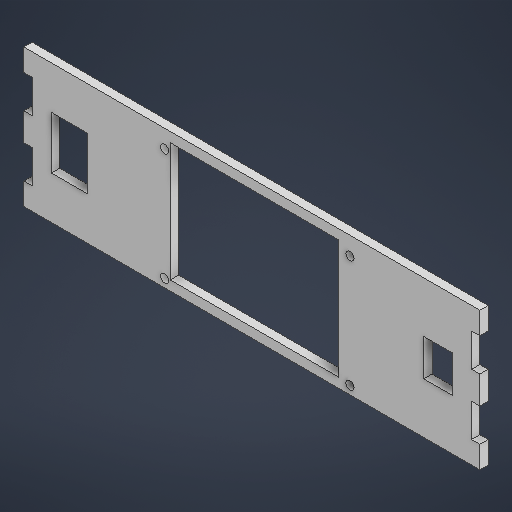
# Autodesk Inventor part: pantallaSoport
Saved by Autodesk Inventor 2026 (Build 300175000, 175)
## iProperties
Created: 2026-04-21
Part Number: pantallaSoport
Material: Generic
Document SubType Name: Modeling
Designer: juana
Density: 1 g/cm^3
Appearance: Default
Author: juana
Autodesk Inventor part; units mm, degrees
ref_plane "YZ Plane" through (0, 0, 0) normal (1, 0, 0) x (0, 1, 0)
ref_plane "XZ Plane" through (0, 0, 0) normal (0, 1, 0) x (-1, 0, 0)
ref_plane "XY Plane" through (0, 0, 0) normal (0, 0, 1) x (1, 0, 0)
sketch "Sketch1" plane through (0, 0, 0) normal (0, 0, 1) x (1, 0, 0)
  line L0 (0, 0) -> (165, 0)
  line L1 (165, 0) -> (165, 50)
  line L2 (165, 50) -> (0, 50)
  line L3 (0, 50) -> (0, 0)
  line L4 (0, 50) -> (3, 50)
  line L5 (3, 50) -> (3, 46.5)
  line L6 (3, 46.5) -> (0, 46.5)
  line L7 (0, 46.5) -> (0, 50)
  line L8 (0, 0) -> (3, 0)
  line L9 (3, 0) -> (3, 3.5)
  line L10 (3, 3.5) -> (0, 3.5)
  line L11 (0, 3.5) -> (0, 0)
  line L12 (82.5, 0) -> (82.5, 50) construction
  line L13 (162, 50) -> (162, 46.5)
  line L14 (162, 46.5) -> (165, 46.5)
  line L15 (162, 0) -> (162, 3.5)
  line L16 (162, 3.5) -> (165, 3.5)
  line L17 (44, 46.5) -> (121, 46.5) construction
  line L18 (121, 46.5) -> (121, 3.5) construction
  line L19 (121, 3.5) -> (44, 3.5) construction
  line L20 (44, 3.5) -> (44, 46.5) construction
  line L21 (53, 46.5) -> (114, 46.5)
  line L22 (114, 46.5) -> (114, 3.5)
  line L23 (114, 3.5) -> (53, 3.5)
  line L24 (53, 3.5) -> (53, 46.5)
  line L25 (3, 0) -> (0, 0)
  line L26 (0, 0) -> (0, 8)
  line L27 (0, 8) -> (3, 8)
  line L28 (3, 8) -> (3, 0)
  line L29 (0, 50) -> (3, 50)
  line L30 (3, 50) -> (3, 42)
  line L31 (3, 42) -> (0, 42)
  line L32 (0, 42) -> (0, 50)
  line L33 (0, 42) -> (3, 42)
  line L34 (3, 42) -> (3, 30)
  line L35 (3, 30) -> (0, 30)
  line L36 (0, 30) -> (0, 42)
  line L37 (3, 8) -> (0, 8)
  line L38 (0, 8) -> (0, 20)
  line L39 (0, 20) -> (3, 20)
  line L40 (3, 20) -> (3, 8)
  line L41 (165, 8) -> (162, 8)
  line L42 (162, 42) -> (165, 42)
  line L43 (162, 42) -> (162, 30)
  line L44 (162, 30) -> (165, 30)
  line L45 (165, 20) -> (162, 20)
  line L46 (162, 20) -> (162, 8)
  point P0 (1.5, 25)
  point P1 (0, 25)
  point P2 (1.5, 3.5)
  point P3 (44, 25)
  point P4 (82.5, 46.5)
  point P5 (1.5, 46.5)
  point P6 (119, 5.5)
  point P7 (119, 44.5)
  point P8 (50.5, 44.5)
  point P9 (50.5, 5.5)
  point P10 (0, 46.5)
  point P11 (0, 3.5)
  point P12 (165, 20)
  point P13 (165, 30)
  point P14 (165, 42)
  dimension "d0" = 165
  dimension "d1" = 50
  dimension "d2" = 3
  dimension "d4" = 21.5
  dimension "d5" = 21.5
  dimension "d6" = 77
  dimension "d7" = 61
  dimension "d8" = 9
  dimension "d9" = 2
  dimension "d10" = 2
  dimension "d11" = 2
  dimension "d12" = 6.5
  dimension "d13" = 2
  dimension "d34" = 8
  dimension "d35" = 8
  dimension "d36" = 12
  dimension "d37" = 12
  constraints: 94 end point, 18 parallel, 15 symmetric about line, 9 horizontal, 9 perpendicular, 7 midpoint, 7 vertical alignment, 6 horizontal alignment, 2 point on line
  measures "d0" distance of L1.end L2.end
  measures "d1" distance of L0.end L1.end
  measures "d2" distance of L5.end L6.end
  measures "d4" distance from line of L10 point (1.5, 25)
  measures "d5" distance from line of L6 point (1.5, 25)
  measures "d6" distance of L17.start L17.end
  measures "d7" distance of L21.start L21.end
  measures "d8" distance between parallel lines of L20 L24
  measures "d9" distance from line of L19 point (119, 5.5)
  measures "d10" distance from line of L17 point (119, 44.5)
  measures "d11" distance from line of L18 point (119, 44.5)
  measures "d12" distance from line of L20 point (50.5, 44.5)
  measures "d13" distance from line of L19 point (50.5, 5.5)
  measures "d34" distance of L27.end L8.end
  measures "d35" distance of L29.end L30.end
  measures "d36" distance of L33.end L34.end
  measures "d37" distance of L39.end L27.end
extrude "Extrusion1" add sketch "Sketch1" along normal blind 3 contours L3 L10 L9 L0 | L9 L28 L40 L39 L3 L35 L34 L30 L5 L2 L13 L14 L1 L42 L43 L44 L45 L46 L41 L16 L15 L0 | L3 L27 L28 L10 | L15 L16 L1 L0 | L3 L6 L30 L31 | L3 L2 L5 L6 | L14 L13 L2 L1
sketch "Sketch2" plane through (0, 0, 3) normal (0, 0, 1) x (1, 0, 0)
  line L0 (53, 46.5) -> (114, 46.5) projected
  line L1 (44, 46.5) -> (121, 46.5)
  line L2 (121, 46.5) -> (121, 0)
  line L3 (121, 0) -> (44, 0)
  line L4 (44, 0) -> (44, 46.5)
  line L5 (165, 50) -> (0, 50) projected
  line L6 (0, 8) -> (0, 0) projected
  point P0 (50.92, 43.5)
  point P1 (50.92, 3)
  point P2 (82.5, 46.5)
  point P3 (82.5, 50)
  point P4 (113, 50)
  point P5 (3, 50)
  point P6 (44, 23.25)
  point P7 (0, 4)
  point P8 (0, 46.5)
  point P9 (0, 3.5)
  point P10 (118, 43.5)
  point P11 (118, 3)
  dimension "d17" = 77
  dimension "d18" = 3
  dimension "d19" = 3
  dimension "d20" = 3
  dimension "d28" = 6.92
  constraints: 8 end point, 4 midpoint, 3 horizontal alignment, 3 vertical alignment, 2 parallel, 1 horizontal, 1 perpendicular, 1 point on line
  measures "d17" distance between parallel lines of L2 L4
  measures "d18" distance from line of L1 point (118, 43.5)
  measures "d19" distance from line of L3 point (118, 3)
  measures "d20" distance from line of L2 point (118, 3)
  measures "d28" distance from line of L4 point (50.92, 3)
hole "Hole1" at (50.92, 43.5, 3) at (50.92, 3, 3) at (118, 3, 3) at (118, 43.5, 3) direction (0, 0, -1) diameter 3 end through all
sketch "Sketch3" plane through (0, 0, 3) normal (0, 0, 1) x (1, 0, 0)
  line L0 (10, 34.5) -> (23, 34.5)
  line L1 (23, 34.5) -> (23, 15.5)
  line L2 (23, 15.5) -> (10, 15.5)
  line L3 (10, 15.5) -> (10, 34.5)
  line L4 (0, 8) -> (0, 0) construction
  line L5 (144.7, 31.65) -> (155, 31.65)
  line L6 (155, 31.65) -> (155, 18.35)
  line L7 (155, 18.35) -> (144.7, 18.35)
  line L8 (144.7, 18.35) -> (144.7, 31.65)
  line L9 (165, 20) -> (165, 30) projected
  line L10 (0, 30) -> (0, 20) projected
  point P0 (10, 25)
  point P1 (0, 46.5)
  point P2 (165, 25)
  point P3 (0, 25)
  point P4 (144.7, 25)
  dimension "d29" = 19
  dimension "d30" = 13
  dimension "d31" = 10
  dimension "d38" = 10.3
  dimension "d39" = 13.3
  dimension "d40" = 10
  constraints: 16 end point, 4 midpoint, 4 parallel, 2 horizontal, 2 horizontal alignment, 2 perpendicular
  measures "d29" distance of L2.end L0.start
  measures "d30" distance of L1.end L2.end
  measures "d31" distance between parallel lines of L4 L3
  measures "d38" distance of L5.start L5.end
  measures "d39" distance of L5.end L6.end
  measures "d40" distance from line of point (165, 25) L6
extrude "Extrusion2" cut sketch "Sketch3" against normal blind 10
body "Solid1"
